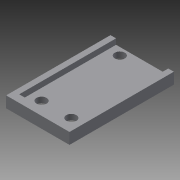
# Autodesk Inventor part: soporte
Saved by Autodesk Inventor 2015 SP1 (Build 190203100, 203)
## iProperties
Created: 2015-06-09
Part Number: soporte
Material: Generic
Document SubType Name: Modeling
Designer: pc
Density: 1 g/cm^3
Appearance: Default
Author: pc
Autodesk Inventor part; units mm, degrees
ref_plane "YZ Plane" through (0, 0, 0) normal (1, 0, 0) x (0, 1, 0)
ref_plane "XZ Plane" through (0, 0, 0) normal (0, 1, 0) x (-1, 0, 0)
ref_plane "XY Plane" through (0, 0, 0) normal (0, 0, 1) x (1, 0, 0)
sketch "Sketch1" plane through (0, 0, 0) normal (0, 0, 1) x (1, 0, 0)
  line L0 (-17, 28) -> (0, 28)
  line L1 (0, 7) -> (0, 0)
  line L2 (0, 0) -> (-17, 0)
  line L3 (-17, 0) -> (-17, 7)
  line L4 (-17, 28) -> (-17, 17)
  line L5 (0, 28) -> (0, 17)
  line L6 (-17, 17) -> (-17, 7)
  line L7 (0, 17) -> (0, 7)
  point P0 (0, 0)
  point P1 (4, 7)
  point P2 (4, 7)
  dimension "d0" = 17
  dimension "d2" = 28
  constraints: 16 end point, 3 vertical, 2 coincident, 2 collinear, 2 perpendicular, 2 other
  measures "d0" distance of L0.start L0.end
  measures "d2" distance between parallel lines of L2 L0
extrude "Extrusion1" add sketch "Sketch1" along normal blind 3
sketch "Sketch2" plane through (0, 0, 3) normal (0, 0, 1) x (1, 0, 0)
  line L0 (-17, 28) -> (-17, 0) projected
  line L1 (-17, 0) -> (0, 0) projected
  line L2 (0, 0) -> (0, 28) projected
  line L3 (0, 28) -> (-17, 28) projected
  line L4 (-17, 0) -> (0, 0) projected
  line L5 (-15.5, 2) -> (-1.5, 2)
  line L6 (-1.5, 2) -> (-1.5, 28)
  line L7 (-1.5, 28) -> (-15.5, 28)
  line L8 (-15.5, 28) -> (-15.5, 2)
  line L9 (0, 28) -> (-17, 28) projected
  dimension "d7" = 14
  dimension "d19" = 26
  constraints: 8 end point, 2 parallel, 1 horizontal, 1 perpendicular, 1 point on line
  measures "d7" distance of L7.end L6.end
  measures "d19" distance of L5.end L6.end
extrude "Extrusion2" cut sketch "Sketch2" against normal blind 1.5 contours L3 L6 L5 L8
sketch "Sketch3" plane through (0, 0, 1.5) normal (0, 0, 1) x (1, 0, 0)
  line L0 (-1.5, 28) -> (-1.5, 2) projected
  line L1 (-15.5, 28) -> (-1.5, 28) projected
  line L2 (-15.5, 2) -> (-15.5, 28) projected
  circle A0 centre (-12.5, 26) radius 1.35
  circle A1 centre (-12.5, 5) radius 1.35
  circle A2 centre (-4.5, 5) radius 1.35
  line L3 (-1.5, 2) -> (-15.5, 2) projected
  point P0 (0, 0)
  dimension "d12" = 2.7
  dimension "d13" = 8
  dimension "d14" = 21
  dimension "d21" = 3
  constraints: 3 centre point, 2 equal radius, 1 horizontal alignment, 1 vertical alignment
  measures "d12" diameter of A1
  measures "d13" distance of A2.centre A1.centre
  measures "d14" distance of A1.centre A0.centre
  measures "d21" distance from line of L3 A1.centre
extrude "Extrusion3" cut sketch "Sketch3" against normal through all contours A0 | A1 | A2
body "Solid1"
